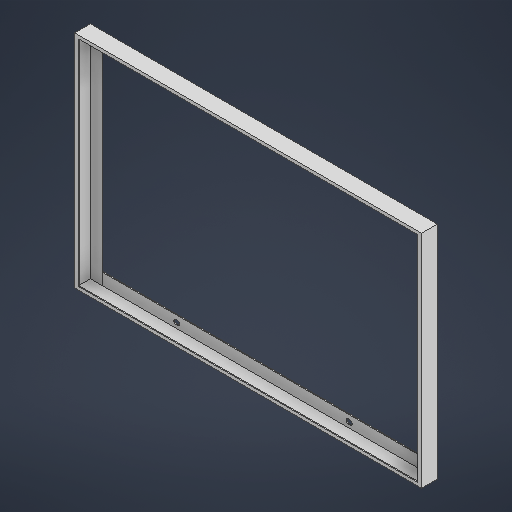
# Autodesk Inventor part: marco
Saved by Autodesk Inventor 2026.2 (Build 302298000, 298)
## iProperties
Created: 2026-01-05
Part Number: marco
Material: Genérico
Document SubType Name: Modeling
Designer: vicho
Density: 1 g/cm^3
Appearance: Valor por defecto
Author: vicho
Autodesk Inventor part; units mm, degrees
ref_plane "YZ Plane" through (0, 0, 0) normal (1, 0, 0) x (0, 1, 0)
ref_plane "XZ Plane" through (0, 0, 0) normal (0, 1, 0) x (-1, 0, 0)
ref_plane "XY Plane" through (0, 0, 0) normal (0, 0, 1) x (1, 0, 0)
sketch "Boceto1" plane through (0, 0, 0) normal (0, 1, 0) x (-1, 0, 0)
  line L0 (867.2697, 0) -> (-1087.5334, 0) construction
  line L1 (0, 1692.3308) -> (0, -1743.0334) construction
  line L2 (-275, -175) -> (275, -175)
  line L3 (275, -175) -> (275, 175)
  line L4 (275, 175) -> (-275, 175)
  line L5 (-275, 175) -> (-275, -175)
  line L6 (-275, -175) -> (275, 175) construction
  line L7 (275, -175) -> (-275, 175) construction
  point P0 (0, 0)
  dimension "d0" = 550
  dimension "d1" = 350
  constraints: 16 end point, 2 horizontal, 2 midpoint, 2 parallel, 2 point on line, 1 perpendicular, 1 vertical
  measures "d0" distance of L4.end L3.end
  measures "d1" distance of L2.end L3.end
extrude "Extrusión1" add sketch "Boceto1" along normal blind 25
sketch "Boceto2" plane through (0, 25, 0) normal (0, 1, 0) x (1, 0, 0)
  line L0 (273.5, 173.5) -> (-273.5, 173.5)
  line L1 (-273.5, 173.5) -> (-273.5, -173.5)
  line L2 (-273.5, -173.5) -> (273.5, -173.5)
  line L3 (273.5, -173.5) -> (273.5, 173.5)
  line L4 (273.5, 173.5) -> (-273.5, -173.5) construction
  line L5 (-273.5, 173.5) -> (273.5, -173.5) construction
  line L6 (-275, 175) -> (-275, -175) projected
  line L7 (-275, -175) -> (275, -175) projected
  point P0 (0, 0)
  dimension "d4" = 1.5
  dimension "d5" = 1.5
  constraints: 12 end point, 2 midpoint, 2 parallel, 1 horizontal, 1 perpendicular
  measures "d4" distance between parallel lines of L6 L1
  measures "d5" distance between parallel lines of L7 L2
extrude "Extrusión2" cut sketch "Boceto2" against normal blind 23.5
sketch "Boceto3" plane through (273.5, 25, 173.5) normal (0, 0, -1) x (-1, 0, 0)
  line L0 (0, 0) -> (547, 0) projected
  line L1 (547, 0) -> (0, 0)
  line L2 (0, 0) -> (0, -1.5)
  line L3 (0, -1.5) -> (546.8806, -1.5)
  line L4 (546.8806, -1.5) -> (547, -1.5)
  line L5 (547, -1.5) -> (547, 0)
  point P0 (273.5, -25)
  dimension "d8" = 1.5
  constraints: 10 end point, 3 perpendicular, 1 collinear, 1 point on line
  measures "d8" distance of L0.start L2.end
extrude "Extrusión3" add sketch "Boceto3" along normal blind 18.5
sketch "Boceto4" plane through (-273.5, 1.5, -173.5) normal (1, 0, 0) x (0, 0, -1)
  line L0 (-328.5, 23.5) -> (0, 23.5) projected
  line L1 (-328.5, 23.5) -> (-328.5, 22) projected
  line L2 (0, 23.5) -> (-328.5, 23.5)
  line L3 (-328.5, 23.5) -> (-328.5, 22)
  line L4 (-328.5, 22) -> (0, 22.0229)
  line L5 (0, 23.5) -> (0, 0) projected
  point P0 (-173.5, -1.5)
  dimension "d11" = 1.5
  constraints: 6 end point, 1 collinear, 1 perpendicular, 1 point on line
  measures "d11" distance of L0.start L1.end
extrude "Extrusión4" add sketch "Boceto4" along normal blind 18.5
sketch "Boceto5" plane through (-273.5, 1.5, -173.5) normal (0, 0, 1) x (1, 0, 0)
  line L0 (548.5, 23.5) -> (-1.5, 23.5) projected
  line L1 (546.9606, 23.5) -> (18.5241, 23.5)
  line L2 (18.5, 23.5) -> (18.5, 22.0229) projected
  line L3 (18.5, 22.0229) -> (547, 22.0229)
  line L4 (547, 23.5) -> (547, 0) projected
  line L5 (547, 23.5) -> (546.9606, 23.5)
  point P0 (273.5, -1.5)
  constraints: 6 end point, 3 point on line, 1 collinear, 1 parallel
extrude "Extrusión5" add sketch "Boceto5" along normal blind 18.5
sketch "Boceto6" plane through (273.5, 1.5, -173.5) normal (-1, 0, 0) x (0, 0, 1)
  line L0 (18.5, 23.5) -> (328.5, 23.5) projected
  line L1 (18.5, 23.5) -> (328.5, 23.5)
  line L2 (328.5, 23.5) -> (328.5, 22.0229)
  line L3 (18.5, 23.5) -> (18.5, 22.0229) projected
  line L4 (328.5, 22.0229) -> (18.5, 22.0229)
  line L5 (18.5, 22.0229) -> (18.5, 23.5)
  point P0 (173.5, -1.5)
  constraints: 8 end point, 3 equal length, 1 perpendicular
extrude "Extrusión6" add sketch "Boceto6" along normal blind 18.5
sketch "Boceto7" plane through (0, 0, 0) normal (0, -1, 0) x (1, 0, 0)
  line L0 (268.5, -170) -> (-268.5, -170)
  line L1 (-268.5, -170) -> (-268.5, 170)
  line L2 (-268.5, 170) -> (268.5, 170)
  line L3 (268.5, 170) -> (268.5, -170)
  line L4 (268.5, -170) -> (-268.5, 170) construction
  line L5 (-268.5, -170) -> (268.5, 170) construction
  line L6 (-275, 175) -> (275, 175) projected
  line L7 (-273.5, 173.5) -> (-273.5, -173.5) projected
  point P0 (0, 0)
  dimension "d18" = 5
  dimension "d19" = 5
  constraints: 12 end point, 2 midpoint, 2 parallel, 1 horizontal, 1 perpendicular
  measures "d18" distance between parallel lines of L6 L2
  measures "d19" distance between parallel lines of L7 L1
extrude "Extrusión7" cut sketch "Boceto7" against normal blind 10
sketch "Boceto8" plane through (0, 25, 0) normal (0, 1, 0) x (1, 0, 0)
  line L0 (-268.5, -170) -> (-268.5, 170) projected
  line L1 (-268.5, 122.5507) -> (-268.5, 115.1946)
  line L2 (-268.5, -170) -> (268.5, -170) projected
  line L3 (-149.9016, -170) -> (-169.2021, -170)
  line L4 (-138, -161.5) -> (-135, -161.5)
  line L5 (-138, -168.5) -> (-135, -168.5)
  arc A0 (-138, -161.5) -> (-138, -168.5) centre (-138, -165) ccw
  arc A1 (-135, -168.5) -> (-135, -161.5) centre (-135, -165) ccw
  line L6 (-255, -155) -> (255, -155) projected
  line L7 (-275, 175) -> (-275, -175) projected
  line L8 (-288.7354, 0) -> (111.6009, 0) construction
  line L9 (0, -308.0533) -> (0, 294.465) construction
  line L10 (138, -161.5) -> (135, -161.5)
  line L11 (138, -168.5) -> (135, -168.5)
  arc A2 (138, -168.5) -> (138, -161.5) centre (138, -165) ccw
  arc A3 (135, -161.5) -> (135, -168.5) centre (135, -165) ccw
  line L12 (288.7354, 0) -> (-111.6009, 0) construction
  line L13 (-138, 161.5) -> (-135, 161.5)
  line L14 (-138, 168.5) -> (-135, 168.5)
  arc A4 (-138, 168.5) -> (-138, 161.5) centre (-138, 165) ccw
  arc A5 (-135, 161.5) -> (-135, 168.5) centre (-135, 165) ccw
  arc A6 (135, 168.5) -> (135, 161.5) centre (135, 165) ccw
  line L15 (138, 161.5) -> (135, 161.5)
  arc A7 (138, 161.5) -> (138, 168.5) centre (138, 165) ccw
  line L16 (138, 168.5) -> (135, 168.5)
  point P0 (0, 0)
  dimension "d22" = 10
  dimension "d23" = 7
  dimension "d24" = 3
  dimension "d25" = 137
  constraints: 26 end point, 20 symmetric about line, 16 point on circle, 8 centre point, 4 horizontal, 4 point on line, 4 tangent, 2 vertical, 6 other
  measures "d22" distance from line of L6 A1.centre
  measures "d23" distance between parallel lines of L4 L5
  measures "d24" distance of A1.centre A0.centre
  measures "d25" distance from line of L7 A0.centre
extrude "Extrusión8" cut sketch "Boceto8" against normal blind 10
